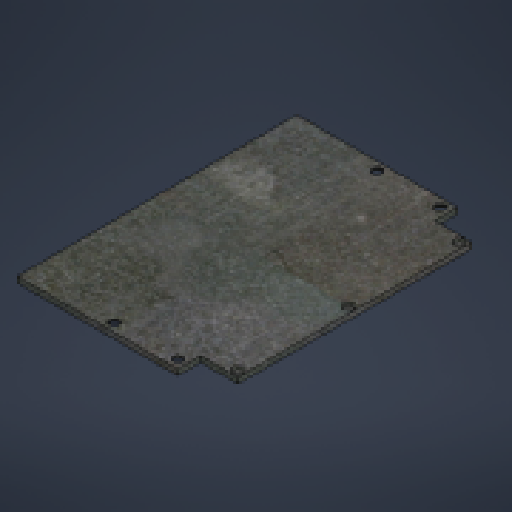
# Autodesk Inventor part: Blacha
Saved by Autodesk Inventor 2023 (Build 270158000, 158)
## iProperties
Created: 2024-01-12
Part Number: Blacha
Material: Steel
Document SubType Name: Modeling
Designer: Michał
Density: 7.85 g/cm^3
Appearance: Plate
Author: Michał
Autodesk Inventor part; units mm, degrees
ref_plane "YZ Plane" through (0, 0, 0) normal (1, 0, 0) x (0, 1, 0)
ref_plane "XZ Plane" through (0, 0, 0) normal (0, 1, 0) x (-1, 0, 0)
ref_plane "XY Plane" through (0, 0, 0) normal (0, 0, 1) x (1, 0, 0)
sketch "Sketch1" plane through (0, 0, 0) normal (0, 1, 0) x (-1, 0, 0)
  line L0 (0, 0) -> (92.5, 0)
  line L1 (92.5, -97.5) -> (0, -97.5)
  line L2 (0, -97.5) -> (0, 0)
  line L3 (92.5, 0) -> (69, 0)
  line L4 (69, 0) -> (69, -97.5)
  line L5 (92.5, -97.5) -> (69, -97.5)
  line L6 (0, -97.5) -> (13, -97.5)
  line L7 (13, -97.5) -> (13, -89.5)
  line L8 (13, -89.5) -> (0, -89.5)
  line L9 (0, -89.5) -> (0, -97.5)
  line L10 (0, 0) -> (13, 0)
  line L11 (13, 0) -> (13, -8)
  line L12 (13, -8) -> (0, -8)
  line L13 (0, -8) -> (0, 0)
  point P0 (69, -97.5)
  dimension "d0" = 92.5
  dimension "d1" = 97.5
  dimension "d4" = 13
  dimension "d5" = 8
  dimension "d24" = 69
  constraints: 28 end point, 5 horizontal, 5 parallel, 3 perpendicular, 1 collinear, 1 point on line
  measures "d0" distance of L1.start L1.end
  measures "d1" distance between parallel lines of L1 L0
  measures "d4" distance between parallel lines of L2 L7
  measures "d5" distance of L6.end L7.end
  measures "d24" distance between parallel lines of L2 L4
extrude "Extrusion1" add sketch "Sketch1" along normal blind 2 contours L0 L4 L1 L7 L8 L2 L12 L11
sketch "Sketch2" plane through (0, 2, 0) normal (0, 1, 0) x (1, 0, 0)
  circle A0 centre (-2.2, 10.15) radius 1.6421 projected
  circle A1 centre (-2.2, 48.75) radius 1.6421 projected
  circle A2 centre (-2.2, 87.35) radius 1.6421 projected
  point P0 (0, 0)
hole "Hole1" at (-2.2, 2, -10.15) at (-2.2, 2, -48.75) at (-2.2, 2, -87.35) direction (0, -1, 0) diameter 2.459 end through all countersink diameter 3.6 countersink angle 90 thread size "M3x0.5" class "6H" standard "ISO Metric profile"
sketch "Sketch3" plane through (0, 0, 0) normal (0, -1, 0) x (1, 0, 0)
  line L0 (-13, -97.5) -> (-69, -97.5) construction
  line L1 (-13, -89.5) -> (-13, -97.5) construction
  line L2 (0, -8) -> (0, -89.5) construction
  line L3 (0, -48.75) -> (-69, -48.75) construction
  line L4 (-69, -97.5) -> (-69, 0) construction
  point P0 (-13, 0)
  point P1 (-16, -94.5)
  point P2 (-38, -94.5)
  point P3 (-16, -3)
  point P4 (-38, -3)
  dimension "d25" = 3
  dimension "d26" = 3
  dimension "d27" = 22
  constraints: 2 end point, 2 midpoint, 2 symmetric about line, 1 horizontal alignment
  measures "d25" distance from line of L0 point (-16, -94.5)
  measures "d26" distance from line of L1 point (-16, -94.5)
  measures "d27" distance of point (-16, -94.5) point (-38, -94.5)
hole "Hole2" at (-16, 0, -94.5) at (-38, 0, -94.5) at (-16, 0, -3) at (-38, 0, -3) direction (0, 1, 0) diameter 3.4 end through all countersink diameter 6.3 countersink angle 90 clearance for "Countersunk Flat Head Screw ISO 2009/7046" size "M3" standard "ISO"
body "Solid1"
